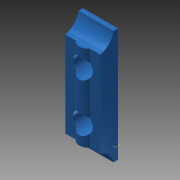
# Autodesk Inventor part: OfflineBowdenExtruderSpringHandle
Saved by Autodesk Inventor 2015 SP1 (Build 190203100, 203)
## iProperties
Created: 2015-04-30
Part Number: OfflineBowdenExtruderSpringHandle
Material: ABS Plastic
Document SubType Name: Modeling
Designer: Jack
Density: 1.06 g/cm^3
Appearance: Cyan
Author: Jack
Autodesk Inventor part; units mm, degrees
ref_plane "YZ Plane" through (0, 0, 0) normal (1, 0, 0) x (0, 1, 0)
ref_plane "XZ Plane" through (0, 0, 0) normal (0, 1, 0) x (-1, 0, 0)
ref_plane "XY Plane" through (0, 0, 0) normal (0, 0, 1) x (1, 0, 0)
sketch "Sketch1" plane through (0, 0, 0) normal (0, 0, 1) x (1, 0, 0)
  line L0 (0, 0) -> (8, 0)
  line L1 (8, 0) -> (8, 4)
  line L2 (8, 4) -> (0, 4)
  line L3 (0, 4) -> (0, 0)
  dimension "d0" = 8
  dimension "d1" = 4
  constraints: 8 end point, 2 parallel, 1 horizontal, 1 perpendicular
  measures "d0" distance of L2.end L1.end
  measures "d1" distance of L1.end L0.end
extrude "Extrusion1" add sketch "Sketch1" along normal blind 26
sketch "Sketch3" plane through (8, 0, 0) normal (1, 0, 0) x (0, 0, -1)
  line L0 (0, 0) -> (0, 4) projected
  line L1 (-26, 0) -> (-26, 4) projected
  line L2 (0, 0) -> (-26, 0) projected
  arc A0 (-22.8, 0) -> (-26, 3) centre (-26.6879, -0.9404) ccw
  arc A1 (0, 3) -> (-3.2, 0) centre (0.6879, -0.9404) ccw
  dimension "d14" = 4
  dimension "d15" = 3.2
  dimension "d16" = 1
  constraints: 4 point on circle, 4 point on line, 2 centre point, 2 horizontal alignment, 1 equal radius
  measures "d14" radius of A0
  measures "d15" distance of L1.start A0.start
  measures "d16" distance of L1.end A0.end
extrude "Extrusion2" cut sketch "Sketch3" against normal up to next
ref_plane "Work Plane1" through (0, 0, 3.2) normal (0, 0, -1) x (-1, 0, 0)
sketch "Sketch4" plane through (0, 0, 3.2) normal (0, 0, -1) x (-1, 0, 0)
  line L0 (0, 0) -> (-8, 0) projected
  line L1 (-8, 0) -> (0, 0) projected
  arc A0 (-5.6, 0) -> (-2.4, 0) centre (-4, 1.2) ccw
  line L2 (-8, 0) -> (-8, 3) projected
  line L3 (-5.6, 0) -> (-2.4, 0)
  dimension "d20" = 2
  dimension "d21" = 4
  dimension "d22" = 1.2
  constraints: 2 end point, 2 point on circle, 2 point on line, 1 centre point, 1 collinear
  measures "d20" radius of A0
  measures "d21" distance from line of L2 A0.centre
  measures "d22" distance from line of L0 A0.centre
extrude "Extrusion3" add sketch "Sketch4" against normal blind 19.6
sketch "Sketch2" plane through (0, 4, 0) normal (0, 1, 0) x (1, 0, 0)
  line L0 (8, -26) -> (0, -26) projected
  line L1 (8, 0) -> (8, -26) projected
  point P0 (4, -7.5)
  point P1 (4, -18.5)
  dimension "d4" = 11
  dimension "d5" = 7.5
  dimension "d6" = 4
  constraints: 1 vertical alignment
  measures "d4" distance of point (4, -18.5) point (4, -7.5)
  measures "d5" distance from line of L0 point (4, -18.5)
  measures "d6" distance from line of L1 point (4, -7.5)
hole "Hole1" at (4, 4, 7.5) at (4, 4, 18.5) direction (0, -1, 0) diameter 4.5 end through all
body "Solid1"
